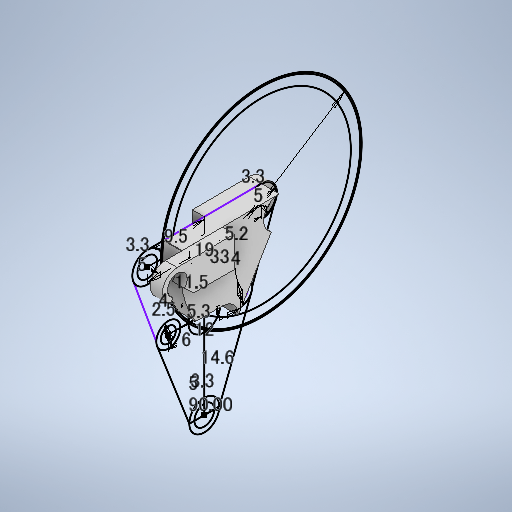
# Autodesk Inventor part: ikafly2c2
Saved by Autodesk Inventor 2025 (Build 290162000, 162)
## iProperties
Created: 2024-06-13
Part Number: ikafly2c2
Material: 一般
Document SubType Name: Modeling
Designer: Saigusa
Density: 1 g/cm^3
Appearance: 既定
Author: Saigusa
Autodesk Inventor part; units mm, degrees
ref_plane "YZ Plane" through (0, 0, 0) normal (1, 0, 0) x (0, 1, 0)
ref_plane "XZ Plane" through (0, 0, 0) normal (0, 1, 0) x (-1, 0, 0)
ref_plane "XY Plane" through (0, 0, 0) normal (0, 0, 1) x (1, 0, 0)
sketch "スケッチ1" plane through (0, 0, 0) normal (1, 0, 0) x (0, 1, 0)
  line L0 (0, 0) -> (0, 6)
  line L1 (0, 6) -> (0, -6)
  line L2 (0, 0) -> (11.5, 0)
  line L3 (11.5, 0) -> (11.5, 9.5)
  line L4 (11.5, 9.5) -> (11.5, -9.5)
  circle A0 centre (0, 6) radius 1.25
  circle A1 centre (0, -6) radius 1.25
  circle A2 centre (11.5, 9.5) radius 1.65
  circle A3 centre (11.5, -9.5) radius 1.65
  circle A4 centre (11.5, 9.5) radius 2.5
  circle A5 centre (11.5, -9.5) radius 2.5
  circle A6 centre (0, 0) radius 2.65
  line L5 (0, 0) -> (-14.6, 0)
  circle A7 centre (-14.6, 0) radius 1.65
  circle A8 centre (-14.6, 0) radius 2.5
  circle A9 centre (0, 6) radius 2
  circle A10 centre (0, -6) radius 2
  line L6 (0, 8) -> (10.6499, 11.851)
  line L7 (0, -8) -> (10.6499, -11.851)
  line L8 (-14.6, 0) -> (-14.6, -2.5)
  line L9 (-14.6, 0) -> (-12.1, 0) construction
  line L10 (-14.6, -2.5) -> (-14.6, 2.5)
  line L11 (-14.6, -2.5) -> (-0.7212, -7.8655)
  line L12 (-14.6, 2.5) -> (-0.7212, 7.8655)
  circle A11 centre (11.5, -9.5) radius 14.9164
  line L13 (11.5, -9.5) -> (0, 0)
  line L14 (11.5, -9.5) -> (0, -2.65)
  line L15 (14, 9.5) -> (14, 6.6979)
  circle A12 centre (11.5, -9.5) radius 16.7294
  circle A13 centre (11.5, -9.5) radius 2.6
  circle A14 centre (11.5, -9.5) radius 16.5
  line L16 (14, 6.6979) -> (14.1, -9.4839)
  line L17 (8.9, -9.5) -> (8.9, 0)
  line L18 (9, 9.5) -> (9, 0)
  line L19 (14.0414, 0) -> (11.5, 0)
  line L20 (0, 2.65) -> (2.65, 2.65)
  line L21 (2.65, 2.65) -> (2.65, 0)
  line L22 (2.65, 2.65) -> (2.65, 4.4258)
  point P0 (9.3522, -8.2206)
  point P1 (0, 2.65)
  point P2 (12.4812, 7.2006)
  point P3 (14, 6.8095)
  point P4 (0.3158, 2.6311)
  point P5 (9.2662, -8.1695)
  dimension "d9" = 5
  dimension "d22" = 33
  dimension "d0" = 6
  dimension "d1" = 12
  dimension "d2" = 11.5
  dimension "d3" = 9.5
  dimension "d4" = 19
  dimension "d5" = 2.5
  dimension "d6" = 3.3
  dimension "d7" = 3.3
  dimension "d8" = 5
  dimension "d10" = 5.3
  dimension "d11" = 14.6
  dimension "d12" = 3.3
  dimension "d13" = 5
  dimension "d14" = 4
  dimension "d15" = 4
  dimension "d16" = 90
  dimension "d21" = 5.2
  constraints: 46 end point, 15 coincident, 14 point on circle, 12 point on line, 11 centre point, 8 tangent, 7 perpendicular, 2 horizontal, 1 parallel, 1 vertical, 13 other
  measures "d0" distance of L0.start L0.end
  measures "d1" distance of L0.end L1.end
  measures "d2" distance of L0.start L2.end
  measures "d3" distance of L2.end L3.end
  measures "d4" distance of L3.end L4.end
  measures "d5" diameter of A0
  measures "d6" diameter of A2
  measures "d7" diameter of A3
  measures "d8" diameter of A4
  measures "d10" diameter of A6
  measures "d11" distance of L5.start L5.end
  measures "d12" diameter of A7
  measures "d13" diameter of A8
  measures "d14" diameter of A9
  measures "d15" diameter of A10
  measures "d16" angle of L8 L9
  measures "d21" diameter of A13
extrude "押し出し3" add sketch "スケッチ1" along normal blind 3 contours A6 L13 L17 L14 | L21 A11 L18 L2 | L2 L17 L13 A6 | L17 L13 A13 L14 | L2 L4 A13 L13 L17 | L21 L22 A14 L18 A11 | L18 A11 L3 L2 | L18 A14 L3 A11 | L19 L16 A13 L4 | L3 A11 L16 L19 | L3 A14 L15 L16 A11
extrude "押し出し4" add sketch "スケッチ1" against normal blind 2 contours L17 L13 A13 L14 | L14 A13 L17 | L2 L4 A13 L13 L17 | A13 L13 A5 L14 | L14 A5 L7 A13 | A13 L4 A5 L13 | L14 A3 L4 A5 | A5 L13 A3 L14 | L7 A5 L4 A13 | L19 L16 A13 L4 | A5 L4 A3 L13
sketch "スケッチ2" plane through (3, 0, 0) normal (1, 0, 0) x (0, 0, -1)
  line L0 (0, 0) -> (0, 11.4707)
  line L1 (0, 14.0414) -> (0, 8.9) projected
  line L2 (0, 11.4707) -> (-9.5, 11.4707)
  circle A0 centre (-9.5, 11.4707) radius 1.65
  circle A1 centre (-9.5, 11.4707) radius 2.5
  line L3 (-9.5186, 8.9708) -> (0, 8.9)
  line L4 (0, 11.4707) -> (0, 14.0414)
  line L5 (0, 14.0414) -> (-6.6979, 14) projected
  line L6 (0, 14.0414) -> (-9.5186, 13.9706)
  line L7 (-9.5, 11.4707) -> (-6.8033, 8.9506)
  line L8 (-9.5, 11.4707) -> (-12, 11.4707)
  line L9 (0, 8.9) -> (7.9513, 8.9) projected
  line L10 (-10.6293, 9.2403) -> (-9.5, 11.4707)
  point P0 (-11.15, 11.4707)
  point P1 (-8.2945, 10.3441)
  point P2 (-10.2453, 9.9986)
  dimension "d27" = 9.5
  dimension "d28" = 3.3
  dimension "d29" = 5
  constraints: 16 end point, 4 point on circle, 2 centre point, 2 coincident, 2 tangent, 1 collinear, 1 midpoint, 1 parallel, 1 perpendicular, 1 point on line
  measures "d27" distance of L0.end L2.end
  measures "d28" diameter of A0
  measures "d29" diameter of A1
extrude "押し出し5" add sketch "スケッチ2" along normal blind 2 contours L3 L7 A1 L2 L0 | L2 A1 L6 L1 | A1 L7 A0 L2 | L2 A0 L8 A1 | A1 L8 A0 L10
